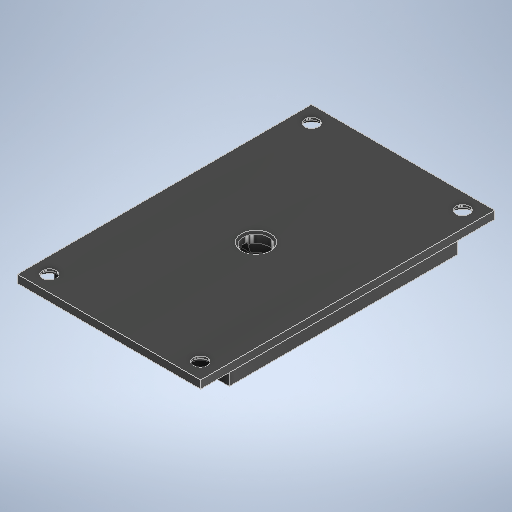
# Autodesk Inventor part: Flex holder Base V1 TPMockup
Saved by Autodesk Inventor 2025 (Build 290162000, 162)
## iProperties
Created: 2025-07-06
Part Number: Flex holder Base V1 TPMockup
Material: Generic
Document SubType Name: Modeling
Designer: Caleb Fangmeier
Density: 1 g/cm^3
Appearance: Dark Gray
Author: Caleb Fangmeier
Autodesk Inventor part; units mm, degrees
ref_plane "YZ Plane" through (0, 0, 0) normal (1, 0, 0) x (0, 1, 0)
ref_plane "XZ Plane" through (0, 0, 0) normal (0, 1, 0) x (-1, 0, 0)
ref_plane "XY Plane" through (0, 0, 0) normal (0, 0, 1) x (1, 0, 0)
sketch "Sketch1" plane through (0, 0, 0) normal (0, 1, 0) x (-1, 0, 0)
  line L0 (-22.05, -28.75) -> (22.05, -28.75)
  line L1 (22.05, -28.75) -> (22.05, 28.75)
  line L2 (22.05, 28.75) -> (-22.05, 28.75)
  line L3 (-22.05, 28.75) -> (-22.05, -28.75)
  line L4 (-22.05, -28.75) -> (22.05, 28.75) construction
  line L5 (22.05, -28.75) -> (-22.05, 28.75) construction
  point P0 (0, 0)
  dimension "d0" = 44.1
  dimension "d1" = 57.5
  constraints: 12 end point, 2 midpoint, 2 parallel, 1 horizontal, 1 perpendicular
  measures "d0" distance of L1.end L2.end
  measures "d1" distance of L0.end L1.end
extrude "Extrusion1" add sketch "Sketch1" along normal blind 2
chamfer "Chamfer1" distance 2 angle 45 1 edges at (-22.05, 1, -28.75)
sketch "Sketch3" plane through (0, 0, 0) normal (0, -1, 0) x (1, 0, 0)
  line L0 (-9.207, 25.75) -> (-19.55, 25.75) construction
  line L1 (-9.207, 24.75) -> (-19.55, 24.75)
  line L2 (-19.55, 26.75) -> (-9.207, 26.75)
  arc A0 (-9.207, 24.75) -> (-9.207, 26.75) centre (-9.207, 25.75) ccw
  arc A1 (-19.55, 26.75) -> (-19.55, 24.75) centre (-19.55, 25.75) ccw
  line L3 (11.239, 25.75) -> (2.834, 25.75) construction
  line L4 (11.239, 26.75) -> (2.834, 26.75)
  line L5 (2.834, 24.75) -> (11.239, 24.75)
  arc A2 (11.239, 24.75) -> (11.239, 26.75) centre (11.239, 25.75) ccw
  arc A3 (2.834, 26.75) -> (2.834, 24.75) centre (2.834, 25.75) ccw
  line L6 (19.55, -25.75) -> (9.039, -25.75) construction
  line L7 (19.55, -24.75) -> (9.039, -24.75)
  line L8 (9.039, -26.75) -> (19.55, -26.75)
  arc A4 (19.55, -26.75) -> (19.55, -24.75) centre (19.55, -25.75) ccw
  arc A5 (9.039, -24.75) -> (9.039, -26.75) centre (9.039, -25.75) ccw
  line L9 (-2.585, -25.75) -> (-10.721, -25.75) construction
  line L10 (-2.585, -24.75) -> (-10.721, -24.75)
  line L11 (-10.721, -26.75) -> (-2.585, -26.75)
  arc A6 (-2.585, -26.75) -> (-2.585, -24.75) centre (-2.585, -25.75) ccw
  arc A7 (-10.721, -24.75) -> (-10.721, -26.75) centre (-10.721, -25.75) ccw
  line L12 (-22.05, 28.75) -> (22.05, 28.75) projected
  line L13 (22.05, 28.75) -> (22.05, -28.75) projected
  line L14 (-22.05, -26.75) -> (-22.05, 28.75) projected
  line L15 (22.05, -28.75) -> (-20.05, -28.75) projected
  point P0 (0, 0)
  point P1 (-14.3785, 25.75)
  point P2 (7.0365, 25.75)
  point P3 (14.2945, -25.75)
  point P4 (-6.653, -25.75)
  dimension "d12" = 1
  dimension "d13" = 3
  dimension "d14" = 10.811
  dimension "d15" = 19.216
  dimension "d16" = 3
  dimension "d17" = 2.5
  dimension "d18" = 12.843
  dimension "d21" = 3
  dimension "d22" = 2.5
  dimension "d23" = 10.511
  dimension "d24" = 11.329
  dimension "d25" = 3
  dimension "d26" = 8.136
  constraints: 32 end point, 16 point on circle, 16 tangent, 8 centre point, 7 parallel, 4 midpoint, 3 equal radius, 1 horizontal
  measures "d12" radius of A1
  measures "d13" distance from line of L12 L3.start
  measures "d14" distance from line of L13 L3.start
  measures "d15" distance from line of L13 L3.end
  measures "d16" distance from line of L12 L0.start
  measures "d17" distance from line of L14 L0.end
  measures "d18" distance from line of L14 L0.start
  measures "d21" distance from line of L15 L6.start
  measures "d22" distance from line of L13 L6.start
  measures "d23" distance of L8.start L8.end
  measures "d24" distance from line of L14 L9.end
  measures "d25" distance from line of L15 L9.end
  measures "d26" distance of L11.start L11.end
extrude "Extrusion2" cut sketch "Sketch3" against normal through all
sketch "Sketch7" plane through (0, 2, 0) normal (0, 1, 0) x (1, 0, 0)
  line L0 (19.55, 24.75) -> (9.039, 24.75) projected
  line L1 (11.039, 24.75) -> (13.039, 24.75)
  line L2 (13.039, 24.75) -> (13.039, -1)
  line L3 (13.039, -1) -> (11.039, -1)
  line L4 (11.039, -1) -> (11.039, 24.75)
  line L5 (-4.585, 24.75) -> (-6.585, 24.75)
  line L6 (-6.585, 24.75) -> (-6.585, -1)
  line L7 (-6.585, -1) -> (-4.585, -1)
  line L8 (-4.585, -1) -> (-4.585, 24.75)
  line L9 (-9.207, -24.75) -> (-19.55, -24.75) projected
  line L10 (-13.207, -24.75) -> (-11.207, -24.75)
  line L11 (-11.207, -24.75) -> (-11.207, 1)
  line L12 (-11.207, 1) -> (-13.207, 1)
  line L13 (-13.207, 1) -> (-13.207, -24.75)
  line L14 (6.834, -24.75) -> (4.834, -24.75)
  line L15 (4.834, -24.75) -> (4.834, 1)
  line L16 (4.834, 1) -> (6.834, 1)
  line L17 (6.834, 1) -> (6.834, -24.75)
  line L18 (13.039, -1) -> (-13.207, -1)
  line L19 (-13.207, -1) -> (-13.207, 1)
  line L20 (-13.207, 1) -> (13.039, 1)
  line L21 (13.039, 1) -> (13.039, -1)
  line L22 (-10.721, 26.75) -> (-2.585, 26.75) projected
  arc A0 (-10.721, 26.75) -> (-10.721, 24.75) centre (-10.721, 25.75) ccw projected
  line L23 (-2.585, 24.75) -> (-10.721, 24.75) projected
  arc A1 (-2.585, 24.75) -> (-2.585, 26.75) centre (-2.585, 25.75) ccw projected
  arc A2 (19.55, 24.75) -> (19.55, 26.75) centre (19.55, 25.75) ccw projected
  line L24 (9.039, 26.75) -> (19.55, 26.75) projected
  arc A3 (9.039, 26.75) -> (9.039, 24.75) centre (9.039, 25.75) ccw projected
  line L25 (22.05, 28.75) -> (-20.05, 28.75) projected
  line L26 (-22.05, 26.75) -> (-20.05, 28.75) projected
  line L27 (-22.05, 26.75) -> (-22.05, -28.75) projected
  line L28 (-22.05, -28.75) -> (22.05, -28.75) projected
  arc A4 (-19.55, -24.75) -> (-19.55, -26.75) centre (-19.55, -25.75) ccw projected
  line L29 (-9.207, -26.75) -> (-19.55, -26.75) projected
  arc A5 (-9.207, -26.75) -> (-9.207, -24.75) centre (-9.207, -25.75) ccw projected
  arc A6 (2.834, -24.75) -> (2.834, -26.75) centre (2.834, -25.75) ccw projected
  line L30 (2.834, -24.75) -> (11.239, -24.75) projected
  line L31 (11.239, -26.75) -> (2.834, -26.75) projected
  arc A7 (11.239, -26.75) -> (11.239, -24.75) centre (11.239, -25.75) ccw projected
  line L32 (22.05, -28.75) -> (22.05, 28.75) projected
  line L33 (23.05, -37) -> (-23.05, -37)
  line L34 (-23.05, -37) -> (-23.05, 37)
  line L35 (-23.05, 37) -> (23.05, 37)
  line L36 (23.05, 37) -> (23.05, -37)
  line L37 (23.05, -37) -> (-23.05, 37) construction
  line L38 (-23.05, -37) -> (23.05, 37) construction
  line L39 (-6.585, 20.0263) -> (-6.585, 22.0263)
  point P0 (0, 0)
  point P1 (4.834, -1)
  point P2 (-6.585, -1)
  point P3 (-11.207, -1)
  point P4 (-11.207, 1)
  point P5 (-6.585, 1)
  point P6 (-6.585, 24.75)
  point P7 (-4.585, 1)
  point P8 (4.834, 1)
  point P9 (11.039, 1)
  point P10 (13.039, 24.75)
  point P11 (6.834, -1)
  point P12 (-6.585, -1)
  point P13 (-11.207, 1)
  point P14 (4.834, 1)
  dimension "d0" = 44.1
  dimension "d39" = 2
  dimension "d40" = 2
  dimension "d41" = 2
  dimension "d42" = 2
  dimension "d43" = 1
  dimension "d44" = 1
  dimension "d45" = 2
  dimension "d46" = 2
  dimension "d47" = 2
  dimension "d48" = 2
  dimension "d51" = 74
  dimension "d52" = 46.1
  constraints: 54 end point, 12 parallel, 7 point on line, 6 horizontal, 6 perpendicular, 2 midpoint
  measures "d39" distance between parallel lines of L6 L8
  measures "d40" distance between parallel lines of L4 L2
  measures "d41" distance between parallel lines of L13 L11
  measures "d42" distance between parallel lines of L15 L17
  measures "d43" distance from line of L7 point (0, 0)
  measures "d44" distance from line of L16 point (0, 0)
  measures "d45" distance from line of L11 A5.centre
  measures "d46" distance from line of L15 A6.centre
  measures "d47" distance from line of L8 A1.centre
  measures "d48" distance from line of L4 A3.centre
  measures "d51" distance of L33.end L34.end
  measures "d52" distance of L34.end L35.end
extrude "Extrusion6" add sketch "Sketch7" along normal blind 2 contours L32 L28 L27 L26 L25
sketch "Sketch8" plane through (0, 4, 0) normal (0, 1, 0) x (1, 0, 0)
  line L0 (23.05, 28.75) -> (23.05, 37) projected
  line L1 (-23.05, 37) -> (-23.05, -37) projected
  line L2 (23.05, 37) -> (-23.05, 37)
  line L3 (-23.05, 37) -> (-23.05, -37)
  line L4 (-23.05, -37) -> (23.05, -37)
  line L5 (23.05, -37) -> (23.05, 37)
  point P0 (0, 0)
  point P1 (22.05, 28.75)
  point P2 (-23.05, 37)
  point P3 (22.05, 28.75)
  constraints: 8 end point, 2 parallel, 1 horizontal, 1 perpendicular, 1 other
extrude "Extrusion7" add sketch "Sketch8" along normal blind 2
sketch "Sketch9" plane through (0, 4, 0) normal (0, -1, 0) x (1, 0, 0)
  point P0 (0, 0)
  point P1 (19, -33)
  point P2 (-19, -33)
  point P3 (19, 33)
  point P4 (-19, 33)
  dimension "d55" = 66
  dimension "d56" = 38
  dimension "d57" = 33
  dimension "d58" = 19
  constraints: 2 horizontal alignment, 2 vertical alignment
  measures "d55" distance of point (19, 33) point (19, -33)
  measures "d56" distance of point (-19, -33) point (19, -33)
  measures "d57" vertical distance of point (19, 33) point (0, 0)
  measures "d58" horizontal distance of point (19, -33) point (0, 0)
hole "Hole1" at (19, 4, -33) at (-19, 4, -33) at (19, 4, 33) at (-19, 4, 33) direction (0, 1, 0) diameter 3.4 end through all countersink diameter 6.3 countersink angle 90 clearance for "Flat Head Machine Screw" size "M3" standard "Ansi Metric M Profile"
sketch "Sketch10" plane through (0, 6, 0) normal (0, 1, 0) x (1, 0, 0)
  circle A0 centre (0, 0) radius 3.175
  circle A1 centre (-19, 33) radius 1.7 projected
  dimension "d74" = 6.35
  constraints: 1 centre point, 1 coincident
  measures "d74" diameter of A0
extrude "Extrusion8" cut sketch "Sketch10" against normal blind 4 contours A0
chamfer "Chamfer2" distance 1.5 distance2 0.6 2 edges at (0, 2, 3.175) (0, 2, -3.175)
chamfer "Chamfer3" distance 0.5 angle 45 1 edges at (-3.175, 6, 0)
sketch "Sketch11" plane through (0, 0, 0) normal (0, -1, 0) x (1, 0, 0)
  line L0 (-7, 12.5) -> (7, 12.5)
  line L1 (8, 13.5) -> (8, 16.5)
  line L2 (7, 17.5) -> (-7, 17.5)
  line L3 (-8, 16.5) -> (-8, 13.5)
  line L4 (-8, 12.5) -> (8, 17.5) construction
  line L5 (8, 12.5) -> (-8, 17.5) construction
  line L6 (-7, -17.5) -> (7, -17.5)
  line L7 (8, -16.5) -> (8, -13.5)
  line L8 (7, -12.5) -> (-7, -12.5)
  line L9 (-8, -13.5) -> (-8, -16.5)
  line L10 (-8, -17.5) -> (8, -12.5) construction
  line L11 (8, -17.5) -> (-8, -12.5) construction
  arc A0 (8, 16.5) -> (7, 17.5) centre (7, 16.5) ccw
  arc A1 (7, 12.5) -> (8, 13.5) centre (7, 13.5) ccw
  arc A2 (-8, 13.5) -> (-7, 12.5) centre (-7, 13.5) ccw
  arc A3 (-7, 17.5) -> (-8, 16.5) centre (-7, 16.5) ccw
  arc A4 (8, -13.5) -> (7, -12.5) centre (7, -13.5) ccw
  arc A5 (7, -17.5) -> (8, -16.5) centre (7, -16.5) ccw
  arc A6 (-8, -16.5) -> (-7, -17.5) centre (-7, -16.5) ccw
  arc A7 (-7, -12.5) -> (-8, -13.5) centre (-7, -13.5) ccw
  point P0 (0, 0)
  point P1 (0, 15)
  point P2 (0, -15)
  dimension "d78" = 25
  dimension "d79" = 35
  dimension "d81" = 12.5
  dimension "d82" = 16
  dimension "d83" = 17.5
  dimension "d84" = 1
  constraints: 24 end point, 16 point on circle, 16 point on line, 16 tangent, 8 centre point, 7 equal radius, 5 parallel, 4 midpoint, 2 horizontal, 2 perpendicular, 2 vertical alignment
  measures "d78" distance between parallel lines of L0 L8
  measures "d79" distance between parallel lines of L2 L6
  measures "d81" distance from line of point (0, 0) L0
  measures "d82" distance of L4.end L5.end
  measures "d83" distance from line of L2 point (0, 0)
  measures "d84" radius of A0
extrude "Extrusion9" cut sketch "Sketch11" against normal blind 0.8
equation "\"d57\" = 0.5 * d55"
equation "\"d58\" = 0.5 * d56"
equation "\"d81\" = 0.5 * d78"
equation "\"d83\" = 0.5 * d79"
body "Solid1"
